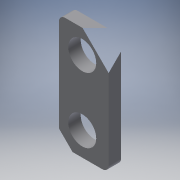
# Autodesk Inventor part: TailConnector2
Saved by Autodesk Inventor 2016 (Build 200138000, 138)
## iProperties
Created: 2017-03-10
Part Number: TailConnector2
Material: Generic
Document SubType Name: Modeling
Designer: Owner
Density: 1 g/cm^3
Appearance: Default
Author: Owner
Autodesk Inventor part; units mm, degrees
ref_plane "YZ Plane" through (0, 0, 0) normal (1, 0, 0) x (0, 1, 0)
ref_plane "XZ Plane" through (0, 0, 0) normal (0, 1, 0) x (-1, 0, 0)
ref_plane "XY Plane" through (0, 0, 0) normal (0, 0, 1) x (1, 0, 0)
sketch "Sketch1" plane through (0, 0, 0) normal (0, 0, 1) x (1, 0, 0)
  circle A0 centre (0, 0.44) radius 1.5 projected
  line L0 (5.5902, 4.25) -> (-5.5902, 4.25) projected
  line L1 (-5.5902, 4.25) -> (-5.5902, -4.25) projected
  line L2 (-5.5902, -4.25) -> (5.5902, -4.25) projected
  line L3 (5.5902, -4.25) -> (5.5902, 4.25) projected
  circle A1 centre (0, -10.06) radius 1.5 projected
  line L4 (5.5902, -6.25) -> (-5.5902, -6.25) projected
  line L5 (-5.5902, -6.25) -> (-5.5902, -13.87) projected
  line L6 (-5.5902, -13.87) -> (5.5902, -13.87) projected
  line L7 (5.5902, -13.87) -> (5.5902, -6.25) projected
  circle A2 centre (0, 0.44) radius 2.25
  circle A3 centre (0, -10.06) radius 2.25
  line L8 (2.25, 4.25) -> (4.25, 4.25)
  line L9 (4.25, 4.25) -> (-3.75, 4.25)
  line L10 (0, -10.06) -> (0, -13.87)
  line L11 (4.25, 4.25) -> (4.25, -13.87)
  line L12 (4.25, -13.87) -> (-3.75, -13.87)
  line L13 (-3.75, -13.87) -> (-3.75, 4.25)
  point P0 (0, 0)
  dimension "d0" = 4.5
  dimension "d1" = 4.5
  dimension "d2" = 2
  dimension "d3" = 8
  constraints: 12 end point, 5 point on line, 2 centre point, 2 coincident, 2 perpendicular, 1 midpoint
  measures "d0" diameter of A2
  measures "d1" diameter of A3
  measures "d2" distance of L8.start L8.end
  measures "d3" distance of L8.end L9.end
extrude "Extrusion1" add sketch "Sketch1" along normal blind 2 contours L11 L2 L13 L0 | L11 L4 L13 L2 | L11 L6 L13 L4
fillet "Fillet1" radius 1 4 edges at (-3.75, -13.87, 1) (-3.75, 4.25, 1) (4.25, -13.87, 1) (4.25, 4.25, 1)
body "Solid1"
